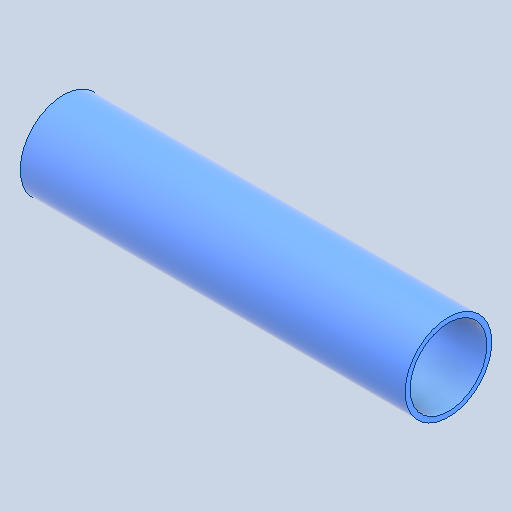
# Autodesk Inventor part: SP001
Saved by Autodesk Inventor 2023 (Build 270158000, 158)
## iProperties
Created: 2022-08-21
Part Number: SP001
Material: PVC, Unplasticized
Document SubType Name: Modeling
Designer: D.C. Eksteen
Mass: 701.904 g
Surface Area: 2160.98 cm^2
Volume: 544.111 cm^3
Density: 1.29 g/cm^3
Appearance: Smooth - White
Authority: 22623906
Description: ROLLER TUBE - CLASS 12 PVC
Author: D.C. Eksteen
Title: ROLLER TUBE
Autodesk Inventor part; units mm, degrees
ref_plane "YZ Plane" through (0, 0, 0) normal (1, 0, 0) x (0, 1, 0)
ref_plane "XZ Plane" through (0, 0, 0) normal (0, 1, 0) x (-1, 0, 0)
ref_plane "XY Plane" through (0, 0, 0) normal (0, 0, 1) x (1, 0, 0)
sketch "Sketch1" plane through (0, 0, 0) normal (1, 0, 0) x (0, 1, 0)
  circle A0 centre (0, 0) radius 45
  circle A1 centre (0, 0) radius 39.9
  dimension "d0" = 90
  dimension "d1" = 5.1
  constraints: 2 centre point, 1 coincident
  measures "d0" diameter of A0
  measures "d1" radial gap between concentric circles of A0 A1
extrude "Extrusion1" add sketch "Sketch1" along normal blind 400
body "Solid1"
